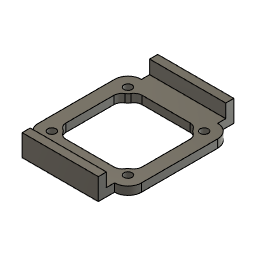
Spacer v2 (Autodesk Fusion 360 design; units mm, degrees)
Autodesk Fusion 360 part; units mm, degrees
note: some values were not read from the file. Set by a fixed rule: which sketch regions a step uses.
sketch "Sketch1" plane through (0, 0, 0) normal (0, 1, 0) x (1, 0, 0)
  circle A0 centre (0, 0) radius 1.5
  circle A1 centre (-28.2, 0) radius 1.5
  circle A2 centre (-28.2, 28.2) radius 1.5
  circle A3 centre (0, 28.2) radius 1.5
  line L0 (-28.2, 23.0038) -> (-28.2, 5.1962)
  line L1 (-23.0038, 0) -> (-5.1962, 0)
  line L2 (0, 23.0038) -> (0, 5.1962)
  line L3 (-5.1962, 28.2) -> (-23.0038, 28.2)
  arc A4 (-26.7, 25.6019) -> (-25.6019, 26.7) centre (-28.2, 28.2) ccw
  arc A5 (-25.6019, 1.5) -> (-26.7, 2.5981) centre (-28.2, 0) ccw
  arc A6 (-1.5, 2.5981) -> (-2.5981, 1.5) centre (0, 0) ccw
  arc A7 (-2.5981, 26.7) -> (-1.5, 25.6019) centre (0, 28.2) ccw
  arc A8 (-26.7, 25.6019) -> (-28.2, 23.0038) centre (-25.2, 23.0038) ccw
  arc A9 (-23.0038, 28.2) -> (-25.6019, 26.7) centre (-23.0038, 25.2) ccw
  arc A10 (-28.2, 5.1962) -> (-26.7, 2.5981) centre (-25.2, 5.1962) ccw
  arc A11 (-25.6019, 1.5) -> (-23.0038, 0) centre (-23.0038, 3) ccw
  arc A12 (-5.1962, 0) -> (-2.5981, 1.5) centre (-5.1962, 3) ccw
  arc A13 (-1.5, 2.5981) -> (0, 5.1962) centre (-3, 5.1962) ccw
  arc A14 (0, 23.0038) -> (-1.5, 25.6019) centre (-3, 23.0038) ccw
  arc A15 (-2.5981, 26.7) -> (-5.1962, 28.2) centre (-5.1962, 25.2) ccw
  arc A16 (-33.2, 0) -> (-28.2, -5) centre (-28.2, 0) ccw
  line L4 (-33.2, 0) -> (-33.2, 28.2)
  arc A17 (-28.2, 33.2) -> (-33.2, 28.2) centre (-28.2, 28.2) ccw
  arc A18 (5, 28.2) -> (0, 33.2) centre (0, 28.2) ccw
  line L5 (5, 28.2) -> (5, 0)
  arc A19 (0, -5) -> (5, 0) centre (0, 0) ccw
  line L6 (-28.2, -11) -> (0, -11)
  line L7 (0, -11) -> (0, -5)
  line L8 (-28.2, -5) -> (-28.2, -11)
  line L9 (-28.2, 39.2) -> (0, 39.2)
  line L10 (0, 39.2) -> (0, 33.2)
  line L11 (-28.2, 33.2) -> (-28.2, 39.2)
  dimension "d1" = 28.2
  dimension "d2" = 28.2
  dimension "d3" = 3
  dimension "d4" = 3
  dimension "d5" = 3
  dimension "d6" = 3
  dimension "d11" = 3
  constraint coincident A0.centre A6.centre
  constraint vertical L0
  constraint perpendicular L0 L1
  constraint perpendicular L1 L2
  constraint perpendicular L2 L3
  constraint tangent L0 A8
  constraint tangent A4 A8
  constraint tangent L3 A9
  constraint tangent A4 A9
  constraint equal A8 A9
  constraint tangent L0 A10
  constraint tangent A5 A10
  constraint equal A8 A10
  constraint tangent L1 A11
  constraint tangent A5 A11
  constraint equal A8 A11
  constraint tangent L1 A12
  constraint tangent A6 A12
  constraint equal A8 A12
  constraint tangent L2 A13
  constraint tangent A6 A13
  constraint equal A8 A13
  constraint tangent L2 A14
  constraint tangent A7 A14
  constraint equal A8 A14
  constraint tangent L3 A15
  constraint tangent A7 A15
  constraint equal A8 A15
  constraint tangent L5 A19
  constraint tangent A16 L4
  constraint tangent L4 A17
  constraint tangent A18 L5
  measures "d1" distance of A0.centre A1.centre
  measures "d2" distance of A0.centre A3.centre
  measures "d3" diameter of A0
  measures "d4" diameter of A1
  measures "d5" diameter of A2
  measures "d6" diameter of A3
  measures "d11" radius of A8
extrude "Extrude1" add sketch "Sketch1" along normal blind 3
sketch "Sketch2" plane through (0, 3, 0) normal (0, 1, 0) x (-1, 0, 0)
  arc A0 (33.2, 0) -> (28.2, 5) centre (28.2, 0) ccw
  line L0 (28.2, 5) -> (28.2, 11)
  line L1 (28.2, 11) -> (0, 11)
  line L2 (0, 11) -> (0, 5)
  arc A1 (0, 5) -> (-5, 0) centre (0, 0) ccw
  line L3 (-5, 0) -> (-5, -28.2)
  arc A2 (-5, -28.2) -> (0, -33.2) centre (0, -28.2) ccw
  line L4 (0, -33.2) -> (0, -39.2)
  line L5 (0, -39.2) -> (28.2, -39.2)
  line L6 (28.2, -39.2) -> (28.2, -33.2)
  arc A3 (28.2, -33.2) -> (33.2, -28.2) centre (28.2, -28.2) ccw
  line L7 (33.2, -28.2) -> (33.2, 0)
  circle A4 centre (0, 0) radius 1.5
  circle A5 centre (28.2, 0) radius 1.5
  circle A6 centre (28.2, -28.2) radius 1.5
  circle A7 centre (0, -28.2) radius 1.5
  line L8 (0, -23.0038) -> (0, -5.1962)
  arc A8 (1.5, -2.5981) -> (0, -5.1962) centre (3, -5.1962) ccw
  arc A9 (1.5, -2.5981) -> (2.5981, -1.5) centre (0, 0) ccw
  arc A10 (5.1962, 0) -> (2.5981, -1.5) centre (5.1962, -3) ccw
  line L9 (5.1962, 0) -> (23.0038, 0)
  arc A11 (25.6019, -1.5) -> (23.0038, 0) centre (23.0038, -3) ccw
  arc A12 (25.6019, -1.5) -> (26.7, -2.5981) centre (28.2, 0) ccw
  arc A13 (28.2, -5.1962) -> (26.7, -2.5981) centre (25.2, -5.1962) ccw
  line L10 (28.2, -5.1962) -> (28.2, -23.0038)
  arc A14 (26.7, -25.6019) -> (28.2, -23.0038) centre (25.2, -23.0038) ccw
  arc A15 (26.7, -25.6019) -> (25.6019, -26.7) centre (28.2, -28.2) ccw
  arc A16 (23.0038, -28.2) -> (25.6019, -26.7) centre (23.0038, -25.2) ccw
  line L11 (23.0038, -28.2) -> (5.1962, -28.2)
  arc A17 (2.5981, -26.7) -> (5.1962, -28.2) centre (5.1962, -25.2) ccw
  arc A18 (2.5981, -26.7) -> (1.5, -25.6019) centre (0, -28.2) ccw
  arc A19 (0, -23.0038) -> (1.5, -25.6019) centre (3, -23.0038) ccw
  line L12 (28.2, -39.2) -> (0, -39.2)
  line L13 (0, -39.2) -> (0, -36.2)
  line L14 (0, -36.2) -> (28.2, -36.2)
  line L15 (28.2, -36.2) -> (28.2, -39.2)
  line L16 (28.2, 11) -> (0, 11)
  line L17 (0, 11) -> (0, 8)
  line L18 (0, 8) -> (28.2, 8)
  line L19 (28.2, 8) -> (28.2, 11)
  dimension "d15" = 3
  dimension "d16" = 3
  constraint horizontal L12
  constraint vertical L13
  constraint horizontal L14
  constraint vertical L15
  constraint coincident L5.end L6.start
  constraint horizontal L16
  constraint vertical L17
  constraint horizontal L18
  constraint vertical L19
  constraint coincident L0.end L1.start
  measures "d15" distance of L5.end L14.end
  measures "d16" distance of L0.end L18.end
extrude "Extrude2" add sketch "Sketch2" along normal blind 5 contours L0 L1 L2 L16 L17 L18 L19 | L4 L5 L6 L12 L13 L14 L15
